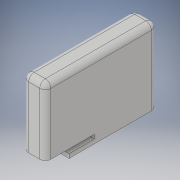
# Autodesk Inventor part: GATE servo motor
Saved by Autodesk Inventor 2017 (Build 210142000, 142)
## iProperties
Created: 2017-03-10
Part Number: GATE servo motor
Material: Generic
Document SubType Name: Modeling
Designer: vitor
Density: 1 g/cm^3
Appearance: Default
Author: vitor
Autodesk Inventor part; units mm, degrees
ref_plane "YZ Plane" through (0, 0, 0) normal (1, 0, 0) x (0, 1, 0)
ref_plane "XZ Plane" through (0, 0, 0) normal (0, 1, 0) x (-1, 0, 0)
ref_plane "XY Plane" through (0, 0, 0) normal (0, 0, 1) x (1, 0, 0)
sketch "Sketch1" plane through (0, 0, 0) normal (1, 0, 0) x (0, 1, 0)
  line L0 (29.3798, 20) -> (5.3798, 20)
  line L1 (5.3798, 20) -> (5.3798, -20)
  line L2 (5.3798, -20) -> (29.3798, -20)
  line L3 (29.3798, -20) -> (29.3798, 20)
  line L4 (5.3798, -20) -> (2.3798, -20)
  line L5 (2.3798, -20) -> (2.3798, 2.5)
  line L6 (2.3798, 2.5) -> (5.3798, 2.5)
  line L7 (5.3798, 2.5) -> (5.3798, -20)
  line L8 (2.3798, 2.5) -> (3.8798, 2.5)
  line L9 (3.8798, 2.5) -> (3.8798, 11.5)
  line L10 (3.8798, 11.5) -> (2.3798, 11.5)
  line L11 (2.3798, 11.5) -> (2.3798, 2.5)
  point P0 (0, 0)
  point P1 (5.3798, 0)
  dimension "d0" = 24
  dimension "d1" = 40
  dimension "d2" = 3
  dimension "d3" = 22.5
  dimension "d4" = 1.5
  dimension "d5" = 9
  constraints: 24 end point, 6 parallel, 3 horizontal, 3 perpendicular, 1 horizontal alignment, 1 midpoint
  measures "d0" distance of L2.end L1.end
  measures "d1" distance of L1.end L0.end
  measures "d2" distance of L5.end L6.end
  measures "d3" distance of L4.end L5.end
  measures "d4" distance of L10.end L9.end
  measures "d5" distance of L9.end L8.end
extrude "Extrusion1" add sketch "Sketch1" along normal blind 8
fillet "Fillet1" radius 2 7 edges at (0, 17.3798, 20) (8, 17.3798, 20) (0, 15.8798, -20) (8, 15.8798, -20) (4, 2.3798, -20) (4, 29.3798, -20) (4, 29.3798, 20)
fillet "Fillet2" radius 2 6 edges at (7.4142, 28.794, 19.4142) (7.4142, 28.794, -19.4142) (8, 29.3798, 0) (0.5858, 28.794, 19.4142) (0.5858, 28.794, -19.4142) (0, 29.3798, 0)
body "Solid1"
